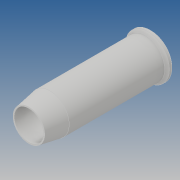
# Autodesk Inventor part: douille
Saved by Autodesk Inventor 2019 (Build 230136000, 136)
## iProperties
Created: 2019-03-23
Part Number: douille
Material: Générique
Document SubType Name: Modeling
Designer: Theo
Density: 1 g/cm^3
Appearance: Par défaut
Author: Theo
Autodesk Inventor part; units mm, degrees
ref_plane "YZ Plane" through (0, 0, 0) normal (1, 0, 0) x (0, 1, 0)
ref_plane "XZ Plane" through (0, 0, 0) normal (0, 1, 0) x (-1, 0, 0)
ref_plane "XY Plane" through (0, 0, 0) normal (0, 0, 1) x (1, 0, 0)
sketch "Esquisse1" plane through (0, 0, 0) normal (1, 0, 0) x (0, 1, 0)
  line L0 (0, 0) -> (0, -31.4318)
  line L1 (6.5, 0) -> (6, 0)
  line L2 (6, 0) -> (6, -50)
  line L3 (6.5, 0) -> (8, -8.5069)
  line L4 (8, -8.5069) -> (8, -48)
  line L5 (6, -50) -> (9, -50)
  line L6 (9, -50) -> (9, -48)
  line L7 (9, -48) -> (8, -48)
  dimension "d0" = 12
  dimension "d1" = 0.5
  dimension "d2" = 170
  dimension "d3" = 50
  dimension "d5" = 16
  dimension "d8" = 2
  dimension "d11" = 1
  dimension "d15" = 3
  constraints: 16 end point, 4 vertical, 3 horizontal, 1 horizontal alignment
  measures "d0" diameter of L2 L0
  measures "d1" distance of L1.start L1.end
  measures "d2" angle of L4 L3
  measures "d3" distance between parallel lines of L1 L5
  measures "d5" diameter of L4 L0
  measures "d8" distance of L5.end L6.end
  measures "d11" distance of L6.end L4.end
  measures "d15" distance between parallel lines of L2 L6
revolve "Révolution1" add sketch "Esquisse1" angle 360 about axis through (0, 0, 0) along (0, 0, -1)
chamfer "Chanfrein1" distance 0.5 angle 45 4 edges at (0, -8, -48) (0, -9, -48) (0, -9, -50) (0, -6, -50)
